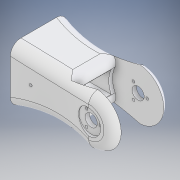
# Autodesk Inventor part: AA010
Saved by Autodesk Inventor 2017 SP1 (Build 210196100, 196)
## iProperties
Created: 2017-09-29
Part Number: AA010
Material: ABS Plastic
Document SubType Name: Modeling
Designer: Zach
Density: 1.06 g/cm^3
Appearance: CR White
Author: Zach
Autodesk Inventor part; units mm, degrees
ref_plane "YZ Plane" through (0, 0, 0) normal (1, 0, 0) x (0, 1, 0)
ref_plane "XZ Plane" through (0, 0, 0) normal (0, 1, 0) x (-1, 0, 0)
ref_plane "XY Plane" through (0, 0, 0) normal (0, 0, 1) x (1, 0, 0)
sketch "Sketch1" plane through (0, 0, 0) normal (0, 0, 1) x (1, 0, 0)
  line L0 (0, 0) -> (0, 105)
  circle A0 centre (32.4, 52.5) radius 2.5
  circle A1 centre (145, 52.5) radius 11.25
  circle A2 centre (145, 52.5) radius 47.5 construction
  arc A3 (145, 5) -> (0, 0) centre (84.2999, -339.6962) ccw
  arc A4 (0, 105) -> (145, 100) centre (84.2999, 444.6962) ccw
  arc A5 (145, 5) -> (145, 100) centre (145, 52.5) ccw
  point P0 (0, 52.5)
  dimension "d0" = 105
  dimension "d1" = 5
  dimension "d2" = 22.5
  dimension "d3" = 112.6
  dimension "d4" = 95
  dimension "d5" = 145
  dimension "d6" = 350
  dimension "d7" = 350
  constraints: 8 point on circle, 6 centre point, 2 end point, 2 horizontal alignment, 2 vertical alignment, 1 coincident, 1 concentric, 1 midpoint, 1 vertical
  measures "d0" distance of L0.start L0.end
  measures "d1" diameter of A0
  measures "d2" diameter of A1
  measures "d3" distance of A1.centre A0.centre
  measures "d4" diameter of A2
  measures "d5" distance of point (0, 52.5) A2.centre
  measures "d6" radius of A3
  measures "d7" radius of A4
extrude "Extrusion1" add sketch "Sketch1" along normal blind 105
sketch "Sketch2" plane through (0, 0, 0) normal (0, 1, 0) x (-1, 0, 0)
  line L0 (0, 0) -> (-145, 0) projected
  arc A0 (0, 0) -> (-145, 0) centre (-72.5, -342.4087) ccw
  line L1 (-145, 105) -> (0, 105) projected
  arc A1 (-145, 105) -> (0, 105) centre (-72.5, 447.4087) ccw
  dimension "d10" = 350
  dimension "d11" = 350
  constraints: 4 point on circle, 2 centre point
  measures "d10" radius of A0
  measures "d11" radius of A1
extrude "Extrusion2" cut sketch "Sketch2" along normal through all
ref_plane "Work Plane1" through (0, 0, 52.5) normal (0, 0, 1) x (1, 0, 0)
sketch "Sketch3" plane through (0, 0, 52.5) normal (0, 0, 1) x (1, 0, 0)
  arc A0 (145, 41.25) -> (145, 63.75) centre (145, 52.5) ccw projected
  arc A1 (145, 41.25) -> (145, 63.75) centre (145, 52.5) ccw projected
  circle A2 centre (145, 52.5) radius 47.5
  point P0 (0, 0)
  dimension "d15" = 95
  constraints: 1 centre point, 1 coincident
  measures "d15" diameter of A2
extrude "Extrusion3" cut sketch "Sketch3" along normal mid plane 79
fillet "Fillet2" radius 15 2 edges at (130.6408, 97.7776, 52.5) (130.6408, 7.2224, 52.5)
fillet "Fillet3" radius 20 4 edges at (71.9844, 94.913, 7.5909) (71.9844, 94.913, 97.4091) (71.9843, 10.087, 97.4091) (71.9843, 10.087, 7.5909)
fillet "Fillet4" radius 20 2 edges at (192.5, 52.5, 105) (192.5, 52.5, 0)
sketch "Sketch4" plane through (0, 19.5779, 105) normal (-1, 0, 0) x (0, 0, 1)
  line L0 (-20, 12.9221) -> (-85, 12.9221)
  line L1 (-85, 12.9221) -> (-85, 52.9221)
  line L2 (-85, 52.9221) -> (-20, 52.9221)
  line L3 (-20, 52.9221) -> (-20, 12.9221)
  line L4 (-85.5772, -19.5779) -> (-19.4228, -19.5779) projected
  line L5 (-105, 0) -> (-105, 65.8443) projected
  point P0 (-105, -19.5779)
  point P1 (-52.5, 12.9221)
  point P2 (-52.5, -19.5779)
  point P3 (-85, 32.9221)
  point P4 (-105, 32.9221)
  dimension "d21" = 65
  dimension "d22" = 40
  constraints: 8 end point, 4 midpoint, 2 parallel, 1 horizontal, 1 horizontal alignment, 1 perpendicular, 1 vertical alignment
  measures "d21" distance of L1.end L2.end
  measures "d22" distance of L0.end L1.end
extrude "Extrusion4" cut sketch "Sketch4" against normal through all
sketch "Sketch5" plane through (0, 19.5779, 105) normal (-1, 0, 0) x (0, 0, 1)
  circle A0 centre (-52.5, 32.9221) radius 39
  line L0 (-85.5772, -19.5779) -> (-19.4228, -19.5779) projected
  line L1 (-105, 0) -> (-105, 65.8443) projected
  point P0 (-105, -19.5779)
  point P1 (-52.5, -19.5779)
  point P2 (-105, 32.9221)
  dimension "d25" = 78
  constraints: 2 midpoint, 1 centre point, 1 horizontal alignment, 1 vertical alignment
  measures "d25" diameter of A0
extrude "Extrusion5" cut sketch "Sketch5" against normal blind 20
sketch "Sketch6" plane through (0, 0, 0) normal (0, 0, -1) x (-1, 0, 0)
  circle A0 centre (-145, 52.5) radius 22.5
  arc A1 (-145, 63.75) -> (-145, 41.25) centre (-145, 52.5) ccw projected
  point P0 (0, 0)
  dimension "d28" = 45
  constraints: 1 centre point, 1 concentric
  measures "d28" diameter of A0
extrude "Extrusion6" cut sketch "Sketch6" against normal blind 5
sketch "Sketch7" plane through (0, 0, 105) normal (0, 0, 1) x (1, 0, 0)
  circle A0 centre (145, 52.5) radius 22.5
  arc A1 (145, 41.25) -> (145, 63.75) centre (145, 52.5) ccw projected
  point P0 (0, 0)
  dimension "d31" = 45
  constraints: 1 centre point, 1 concentric
  measures "d31" diameter of A0
extrude "Extrusion7" cut sketch "Sketch7" against normal blind 5
sketch "Sketch8" plane through (145, 52.5, 100) normal (0, 0, 1) x (1, 0, 0)
  circle A0 centre (17, 0) radius 2.5
  circle A1 centre (0, 0) radius 11.25 construction
  circle A2 centre (-8.5, 14.7224) radius 2.5
  circle A3 centre (-8.5, -14.7224) radius 2.5
  point P0 (-145, -52.5)
  dimension "d34" = 5
  dimension "d35" = 17
  dimension "d38" = 360
  constraints: 3 centre point, 1 horizontal alignment, 7 other
  measures "d34" diameter of A0
  measures "d35" distance of A0.centre A1.centre
extrude "Extrusion8" cut sketch "Sketch8" against normal through all
body "Solid1"
